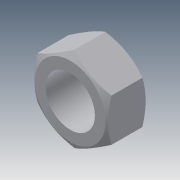
# Autodesk Inventor part: 375 nut
Saved by Autodesk Inventor 2014 (Build 180170000, 170)
## iProperties
Created: 2016-01-12
Part Number: 375 nut
Material: Generic
Document SubType Name: Modeling
Designer: Paul
Density: 1 g/cm^3
Appearance: Default
Author: Paul
Autodesk Inventor part; units mm, degrees
ref_plane "YZ Plane" through (0, 0, 0) normal (1, 0, 0) x (0, 1, 0)
ref_plane "XZ Plane" through (0, 0, 0) normal (0, 1, 0) x (-1, 0, 0)
ref_plane "XY Plane" through (0, 0, 0) normal (0, 0, 1) x (1, 0, 0)
sketch "Sketch1" plane through (0, 0, 0) normal (0, 0, 1) x (1, 0, 0)
  line L0 (0, 8.2489) -> (7.1437, 4.1244)
  line L1 (7.1437, 4.1244) -> (7.1437, -4.1244)
  line L2 (7.1437, -4.1244) -> (0, -8.2489)
  line L3 (0, -8.2489) -> (-7.1438, -4.1244)
  line L4 (-7.1438, -4.1244) -> (-7.1438, 4.1244)
  line L5 (-7.1438, 4.1244) -> (0, 8.2489)
  point P0 (0, 0)
  point P1 (0, 0)
  dimension "d0" = 14.2875
  constraints: 12 end point, 1 coincident, 13 other
  measures "d0" distance between parallel lines of L1 L4
extrude "Extrusion1" add sketch "Sketch1" along normal blind 7.62
sketch "Sketch2" plane through (0, 0, 7.62) normal (0, 0, 1) x (1, 0, 0)
  circle A0 centre (0, 0) radius 4.7625
  dimension "d3" = 9.525
  constraints: 1 centre point, 1 coincident
  measures "d3" diameter of A0
extrude "Extrusion2" cut sketch "Sketch2" against normal blind 7.62
sketch "Sketch3" plane through (0, 0, 7.62) normal (0, 0, 1) x (1, 0, 0)
  circle A0 centre (0, 0) radius 4.7625 projected
  circle A1 centre (0, 0) radius 6.8161
  constraints: 1 centre point, 1 coincident
extrude "Extrusion3" cut sketch "Sketch3" against normal blind 7.62 draft 60 contours A0 | A1 keep common part
sketch "Sketch4" plane through (0, 0, 0) normal (0, 0, -1) x (-1, 0, 0)
  circle A0 centre (0, 0) radius 4.7625 projected
  circle A1 centre (0, 0) radius 6.8291
  constraints: 1 centre point, 1 coincident
extrude "Extrusion4" cut sketch "Sketch4" against normal blind 7.62 draft 60 contours A0 | A1 keep common part
body "Solid1"
